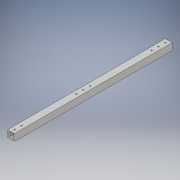
# Autodesk Inventor part: 23in 1x1
Saved by Autodesk Inventor 2018 (Build 220112000, 112)
## iProperties
Created: 2018-12-30
Part Number: 23in 1x1
Material: Generic
Document SubType Name: Modeling
Designer: maste
Density: 1 g/cm^3
Appearance: Default
Author: maste
Autodesk Inventor part; units mm, degrees
ref_plane "YZ Plane" through (0, 0, 0) normal (1, 0, 0) x (0, 1, 0)
ref_plane "XZ Plane" through (0, 0, 0) normal (0, 1, 0) x (-1, 0, 0)
ref_plane "XY Plane" through (0, 0, 0) normal (0, 0, 1) x (1, 0, 0)
sketch "Sketch1" plane through (0, 0, 0) normal (0, 0, 1) x (1, 0, 0)
  line L0 (0, 0) -> (25.4, 0)
  line L1 (25.4, 0) -> (25.4, 25.4)
  line L2 (25.4, 25.4) -> (0, 25.4)
  line L3 (0, 25.4) -> (0, 0)
  line L4 (3.175, 22.225) -> (22.225, 22.225)
  line L5 (22.225, 22.225) -> (22.225, 3.175)
  line L6 (22.225, 3.175) -> (3.175, 3.175)
  line L7 (3.175, 3.175) -> (3.175, 22.225)
  dimension "d0" = 25.4
  dimension "d1" = 25.4
  dimension "d2" = 3.175
  constraints: 16 end point, 4 parallel, 2 perpendicular, 1 horizontal, 3 other
  measures "d0" distance of L2.end L1.end
  measures "d1" distance of L1.end L0.end
  measures "d2" distance between parallel lines of L2 L4
extrude "Extrusion1" add sketch "Sketch1" along normal blind 584.2
sketch "Sketch3" plane through (0, 25.4, 0) normal (0, 1, 0) x (1, 0, 0)
  line L0 (3.175, -584.2) -> (22.225, -584.2) construction
  line L1 (12.7, -584.2) -> (12.7, -304.8) construction
  line L2 (12.7, -304.8) -> (12.7, -317.5) construction
  line L3 (12.7, -317.5) -> (12.7, -342.9) construction
  line L4 (12.7, -342.9) -> (12.7, -292.1) construction
  line L5 (12.7, -584.2) -> (12.7, -571.5) construction
  line L6 (12.7, -571.5) -> (12.7, -546.1) construction
  line L7 (22.225, 0) -> (3.175, 0) construction
  line L8 (12.7, 0) -> (12.7, -12.7) construction
  line L9 (12.7, -12.7) -> (12.7, -38.1) construction
  line L10 (12.7, -38.1) -> (12.7, -63.5) construction
  circle A0 centre (12.7, -12.7) radius 2.5797
  circle A1 centre (12.7, -38.1) radius 2.5797
  circle A2 centre (12.7, -63.5) radius 2.5797
  circle A3 centre (12.7, -317.5) radius 2.5797
  circle A4 centre (12.7, -292.1) radius 2.5797
  circle A5 centre (12.7, -342.9) radius 2.5797
  circle A6 centre (12.7, -546.1) radius 2.5797
  circle A7 centre (12.7, -571.5) radius 2.5797
  point P0 (0, 0)
  dimension "d5" = 279.4
  dimension "d6" = 12.7
  dimension "d7" = 25.4
  dimension "d8" = 50.8
  dimension "d9" = 12.7
  dimension "d10" = 25.4
  dimension "d11" = 12.7
  dimension "d12" = 25.4
  dimension "d13" = 25.4
  dimension "d14" = 5.1594
  constraints: 18 end point, 8 centre point, 8 coincident, 7 point on line, 2 midpoint, 2 vertical
  measures "d5" distance of L1.start L1.end
  measures "d6" distance of L1.end L2.end
  measures "d7" distance of L2.end L3.end
  measures "d8" distance of L3.end L4.end
  measures "d9" distance of L1.start L5.end
  measures "d10" distance of L5.end L6.end
  measures "d11" distance of L8.start L8.end
  measures "d12" distance of L8.end L9.end
  measures "d13" distance of L9.end L10.end
  measures "d14" diameter of A0
extrude "Extrusion2" cut sketch "Sketch3" against normal blind 606.425
body "Solid1"
